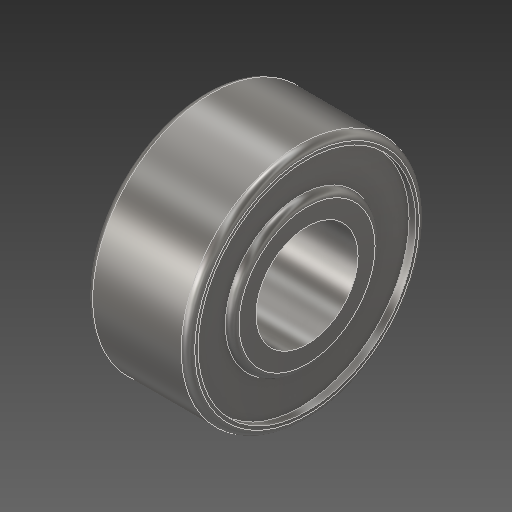
# Autodesk Inventor part: bearing
Saved by Autodesk Inventor 2018 (Build 220112000, 112)
## iProperties
Created: 2018-06-15
Part Number: bearing
Material: 鋼、合金
Document SubType Name: Modeling
Designer: NaMACHAN
Density: 7.73 g/cm^3
Appearance: 半つや出し
Mass: 0.671402 g
Surface Area: 1.64432 cm^2
Volume: 0.0868567 cm^3
Author: NaMACHAN
Autodesk Inventor part; units mm, degrees
ref_plane "YZ Plane" through (0, 0, 0) normal (1, 0, 0) x (0, 1, 0)
ref_plane "XZ Plane" through (0, 0, 0) normal (0, 1, 0) x (-1, 0, 0)
ref_plane "XY Plane" through (0, 0, 0) normal (0, 0, 1) x (1, 0, 0)
sketch "スケッチ1" plane through (0, 0, 0) normal (1, 0, 0) x (0, 1, 0)
  circle A0 centre (0, 0) radius 3.5
  dimension "d0" = 7
  constraints: 1 centre point, 1 coincident
  measures "d0" diameter of A0
extrude "押し出し1" add sketch "スケッチ1" along normal blind 3
sketch "スケッチ2" plane through (3, 0, 0) normal (1, 0, 0) x (0, 0, -1)
  circle A0 centre (0, 0) radius 1.5
  dimension "d3" = 3
  constraints: 1 centre point, 1 coincident
  measures "d3" diameter of A0
extrude "押し出し2" cut sketch "スケッチ2" against normal blind 3
sketch "スケッチ3" plane through (3, 0, 0) normal (1, 0, 0) x (0, 0, -1)
  circle A0 centre (0, 0) radius 3.2
  circle A1 centre (0, 0) radius 2.2
  circle A2 centre (0, 0) radius 3.5 projected
  dimension "d6" = 0.3
  dimension "d7" = 1
  constraints: 2 centre point, 2 coincident
  measures "d6" radial gap between concentric circles of A2 A0
  measures "d7" radial gap between concentric circles of A0 A1
extrude "押し出し3" cut sketch "スケッチ3" against normal blind 0.2 contours A0
sketch "スケッチ4" plane through (0, 0, 0) normal (-1, 0, 0) x (0, 0, 1)
  circle A0 centre (0, 0) radius 3.2 projected
  circle A1 centre (0, 0) radius 2.2 projected
extrude "押し出し4" cut sketch "スケッチ4" against normal blind 0.2
fillet "フィレット1" radius 0.2 4 edges at (0, -3.5, 0) (0, 0, -2.2) (3, -3.5, 0) (3, 0, 2.2)
